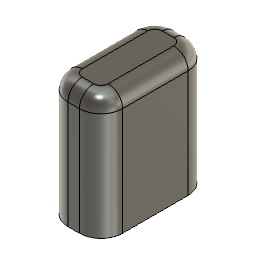
UsbHolder (Autodesk Fusion 360 design; units mm, degrees)
part number: 2026-06-15-18-58-49-807
Autodesk Fusion 360 part; units mm, degrees
sketch "Sketch2" plane through (0, 0, 0) normal (0, 0, 1) x (1, 0, 0)
  line L0 (0, 0) -> (4.6, 0)
  line L1 (4.6, 0) -> (4.6, 12.1)
  line L2 (4.6, 12.1) -> (0, 12.1)
  line L3 (0, 12.1) -> (0, 0)
  line L4 (-1.5, 13.6) -> (6.1, 13.6)
  line L5 (6.1, 13.6) -> (6.1, -1.5)
  line L6 (6.1, -1.5) -> (-1.5, -1.5)
  line L7 (-1.5, -1.5) -> (-1.5, 13.6)
  dimension "d1" = 4.6
  dimension "d2" = 12.1
  dimension "d3" = 1.5
  dimension "d4" = 1.5
  dimension "d5" = 1.5
  dimension "d6" = 1.5
  constraint horizontal L0
  constraint vertical L1
  constraint horizontal L2
  constraint vertical L3
  constraint coincident L0.start L3.end
  constraint horizontal L4
  constraint vertical L5
  constraint horizontal L6
  constraint vertical L7
  measures "d1" distance of L0.start L0.end
  measures "d2" distance of L0.start L2.end
  measures "d3" distance of L1 L5
  measures "d4" distance of L3 L7
  measures "d5" distance of L0 L6
  measures "d6" distance of L2 L4
extrude "Extrude1" add sketch "Sketch2" along normal blind 14
sketch "Sketch3" plane through (0, 0, 14) normal (0, 0, 1) x (-1, 0, 0)
  line L0 (0, 0) -> (0, -12.1)
  line L1 (0, -12.1) -> (-4.6, -12.1)
  line L2 (-4.6, -12.1) -> (-4.6, 0)
  line L3 (-4.6, 0) -> (0, 0)
  line L4 (1.5, 1.5) -> (-6.1, 1.5)
  line L5 (-6.1, 1.5) -> (-6.1, -13.6)
  line L6 (-6.1, -13.6) -> (1.5, -13.6)
  line L7 (1.5, -13.6) -> (1.5, 1.5)
  line L8 (1.5, -13.6) -> (-6.1, -13.6)
  line L9 (-6.1, -13.6) -> (-6.1, 1.5)
  line L10 (-6.1, 1.5) -> (1.5, 1.5)
  line L11 (1.5, 1.5) -> (1.5, -13.6)
  constraint horizontal L8
  constraint vertical L9
  constraint horizontal L10
  constraint vertical L11
  constraint coincident L4.end L5.start
  constraint coincident L6.end L7.start
extrude "Extrude2" add sketch "Sketch3" along normal blind 3 contours L0 L1 L2 L3 | L4 L5 L6 L7 L8 L9 L10 L11
fillet "Fillet1" radius 3 4 edges at (-1.5, 13.6, 8.5) (-1.5, -1.5, 8.5) (6.1, -1.5, 8.5) (6.1, 13.6, 8.5)
fillet "Fillet1" radius 2 4 edges at (6.1, 6.05, 17) (2.3, -1.5, 17) (-1.5, 6.05, 17) (2.3, 13.6, 17)
equation "d4 = d3"
equation "d5 = d4"
equation "d6 = d3"
